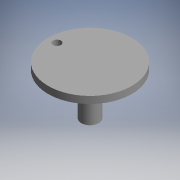
# Autodesk Inventor part: Servo_arm
Saved by Autodesk Inventor 2017 (Build 210142000, 142)
## iProperties
Part Number: Servo_arm
Material: Generic
Document SubType Name: Modeling
Designer: alex-
Appearance: Generic
sa_diameter: 2,400 cm
sa_thickness: 0,200 cm
Author: alex-
Autodesk Inventor part; units mm, degrees
ref_plane "YZ Plane" through (0, 0, 0) normal (1, 0, 0) x (0, 1, 0)
ref_plane "XZ Plane" through (0, 0, 0) normal (0, 1, 0) x (-1, 0, 0)
ref_plane "XY Plane" through (0, 0, 0) normal (0, 0, 1) x (1, 0, 0)
sketch "Sketch1" plane through (0, 0, 0) normal (0, 1, 0) x (-1, 0, 0)
  circle A0 centre (0, 0) radius 12
  dimension "sa_diameter" = 24
  constraints: 1 centre point, 1 coincident
  measures "sa_diameter" diameter of A0
extrude "Extrusion1" add sketch "Sketch1" along normal blind 2
sketch "Sketch2" plane through (0, 0, 0) normal (0, -1, 0) x (1, 0, 0)
  circle A0 centre (0, 0) radius 2.5
  dimension "d4" = 5
  constraints: 1 centre point, 1 coincident
  measures "d4" diameter of A0
extrude "Extrusion2" add sketch "Sketch2" along normal blind 12
sketch "Sketch3" plane through (0, 2, 0) normal (0, 1, 0) x (1, 0, 0)
  circle A0 centre (-9.4812, 0) radius 1.1266
  point P0 (0, 0)
  dimension "d8" = 9.4812
  dimension "d9" = 2.2531
  constraints: 1 centre point, 1 horizontal alignment
  measures "d8" distance of point (0, 0) A0.centre
  measures "d9" diameter of A0
extrude "Extrusion3" cut sketch "Sketch3" against normal up to next
body "Solid1"
